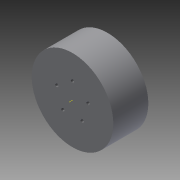
# Autodesk Inventor part: Aluminum mold support
Saved by Autodesk Inventor 2013 (Build 170138000, 138)
## iProperties
Created: 2013-05-10
Part Number: Aluminum mold support
Material: Generic
Document SubType Name: Modeling
Designer: grtstudent
Density: 1 g/cm^3
Author: grtstudent
Autodesk Inventor part; units mm, degrees
ref_plane "YZ Plane" through (0, 0, 0) normal (1, 0, 0) x (0, 1, 0)
ref_plane "XZ Plane" through (0, 0, 0) normal (0, 1, 0) x (-1, 0, 0)
ref_plane "XY Plane" through (0, 0, 0) normal (0, 0, 1) x (1, 0, 0)
sketch "Sketch1" plane through (0, 0, 0) normal (0, 0, 1) x (1, 0, 0)
  circle A0 centre (0, 0) radius 47.371
  dimension "d0" = 94.742
  constraints: 1 centre point, 1 coincident
  measures "d0" diameter of A0
extrude "Extrusion1" add sketch "Sketch1" along normal blind 40.64
sketch "Sketch2" plane through (0, 0, 0) normal (0, 0, -1) x (-1, 0, 0)
  circle A0 centre (0, 0) radius 42.8625
  dimension "d4" = 85.725
  constraints: 1 centre point, 1 coincident
  measures "d4" diameter of A0
extrude "Extrusion2" cut sketch "Sketch2" against normal blind 31.75
sketch "Sketch6" plane through (0, 0, 40.64) normal (0, 0, 1) x (1, 0, 0)
  circle A0 centre (0, 0) radius 47.371 projected
  circle A1 centre (0, 0) radius 19.05
  line L0 (0, 19.05) -> (0, 0) construction
  dimension "d24" = 38.1
  constraints: 2 end point, 1 coincident, 1 vertical, 1 vertical alignment, 2 other
hole "Hole3" at (0, 19.05, 40.64) direction (0, 0, -1) diameter 3.9624 depth 25.4 tip angle 118 thread size "10-32 UNF" class "2B" standard "ANSI Unified Screw Threads"
pattern_circular "Circular Pattern1" count 5 over 360 about axis through (0, 0, 0) along (0, 0, 1) of "Hole3"
body "Solid1"
